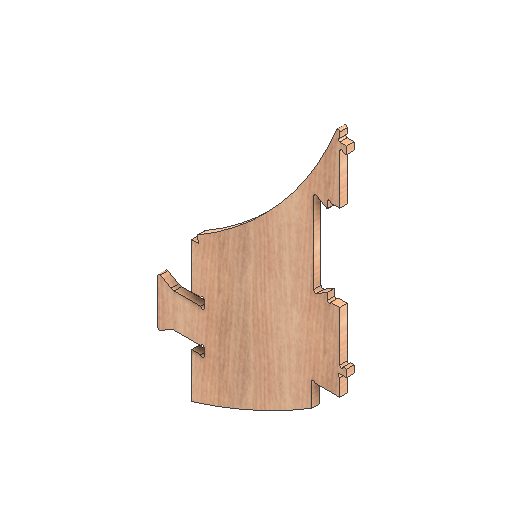
# Autodesk Inventor part: Support B
Saved by Autodesk Inventor 2021 (Build 250183000, 183)
## iProperties
Created: 2020-05-09
Part Number: Support B
Material: Wood (Birch)
Document SubType Name: Modeling
Designer: Dan Wikman
Density: 0.55 g/cm^3
Appearance: Birch - Natural Polished
Mass: 1422.74 g
Surface Area: 3324.08 cm^2
Volume: 2586.8 cm^3
Autodesk Inventor part; units mm, degrees
ref_plane "YZ Plane" through (0, 0, 0) normal (1, 0, 0) x (0, 1, 0)
ref_plane "XZ Plane" through (0, 0, 0) normal (0, 1, 0) x (-1, 0, 0)
ref_plane "XY Plane" through (0, 0, 0) normal (0, 0, 1) x (1, 0, 0)
sketch "CONTOURS" plane through (0, 0, 0) normal (0, 0, 1) x (1, 0, 0)
  line L0 (2379.4087, 421.1241) -> (2379.4087, 437.5136)
  line L1 (2083.0497, 275.5979) -> (2083.0497, 256.5979)
  arc A0 (2075.0497, 256.5979) -> (2083.0497, 256.5979) centre (2079.0497, 256.5979) ccw
  line L2 (2075.0497, 256.5979) -> (2051.9087, 256.5979)
  line L3 (2051.9087, 256.5979) -> (2010.928, 256.5979)
  arc A1 (2003.428, 258.6076) -> (2010.928, 256.5979) centre (2010.928, 271.5979) ccw
  line L4 (2003.428, 258.6076) -> (1977.9087, 273.3411)
  arc A2 (1977.9087, 273.3411) -> (1971.9087, 269.877) centre (1975.9087, 269.877) ccw
  line L5 (1971.9087, 269.877) -> (1971.9087, 161.3189)
  arc A3 (1971.9087, 161.3189) -> (1977.9087, 157.8548) centre (1975.9087, 161.3189) ccw
  line L6 (1977.9087, 157.8548) -> (2003.428, 172.5883)
  arc A4 (2010.928, 174.5979) -> (2003.428, 172.5883) centre (2010.928, 159.5979) ccw
  line L7 (2010.928, 174.5979) -> (2051.9087, 174.5979)
  line L8 (2051.9087, 174.5979) -> (2075.0497, 174.5979)
  arc A5 (2083.0497, 174.5979) -> (2075.0497, 174.5979) centre (2079.0497, 174.5979) ccw
  line L9 (2083.0497, 174.5979) -> (2083.0497, 155.5979)
  arc A6 (2075.0497, 155.5979) -> (2083.0497, 155.5979) centre (2079.0497, 155.5979) ccw
  line L10 (2075.0497, 155.5979) -> (2053.0497, 155.5979)
  line L11 (2053.0497, 155.5979) -> (2053.0497, 46.9498)
  arc A7 (2053.0497, 46.9498) -> (2341.9087, 177.362) centre (1668.415, 1284.0168) ccw
  line L12 (2341.9087, 177.362) -> (2341.9087, 234.1241)
  arc A8 (2349.9087, 234.1241) -> (2341.9087, 234.1241) centre (2345.9087, 234.1241) ccw
  line L13 (2349.9087, 234.1241) -> (2409.4087, 234.1241)
  line L14 (2409.4087, 234.1241) -> (2409.4087, 275.172)
  arc A9 (2409.4087, 283.172) -> (2409.4087, 275.172) centre (2409.4087, 279.172) ccw
  line L15 (2409.4087, 283.172) -> (2425.9087, 283.172)
  line L16 (2425.9087, 283.172) -> (2425.9087, 301.172)
  line L17 (2425.9087, 301.172) -> (2417.4087, 301.172)
  arc A10 (2409.4087, 301.172) -> (2417.4087, 301.172) centre (2413.4087, 301.172) ccw
  line L18 (2409.4087, 301.172) -> (2409.4087, 421.1241)
  line L19 (2409.4087, 421.1241) -> (2387.4087, 421.1241)
  arc A11 (2379.4087, 421.1241) -> (2387.4087, 421.1241) centre (2383.4087, 421.1241) ccw
  line L20 (2379.4087, 437.5136) -> (2379.1671, 437.3833)
  line L21 (2379.1671, 437.3833) -> (2378.928, 437.2484)
  line L22 (2378.928, 437.2484) -> (2353.7677, 422.7221)
  arc A12 (2346.2677, 427.0523) -> (2353.7677, 422.7221) centre (2351.2677, 427.0523) ccw
  line L23 (2346.2677, 427.0523) -> (2346.2677, 622.1959)
  arc A13 (2353.7677, 626.526) -> (2346.2677, 622.1959) centre (2351.2677, 622.1959) ccw
  line L24 (2353.7677, 626.526) -> (2378.928, 611.9997)
  line L25 (2378.928, 611.9997) -> (2379.1671, 611.8648)
  line L26 (2379.1671, 611.8648) -> (2379.4087, 611.7346)
  line L27 (2379.4087, 611.7346) -> (2379.4087, 628.1241)
  arc A14 (2387.4087, 628.1241) -> (2379.4087, 628.1241) centre (2383.4087, 628.1241) ccw
  line L28 (2387.4087, 628.1241) -> (2409.4087, 628.1241)
  line L29 (2409.4087, 628.1241) -> (2409.4087, 748.0761)
  arc A15 (2417.4087, 748.0761) -> (2409.4087, 748.0761) centre (2413.4087, 748.0761) ccw
  line L30 (2417.4087, 748.0761) -> (2425.9087, 748.0761)
  line L31 (2425.9087, 748.0761) -> (2425.9087, 766.0761)
  line L32 (2425.9087, 766.0761) -> (2409.4087, 766.0761)
  arc A16 (2409.4087, 774.0761) -> (2409.4087, 766.0761) centre (2409.4087, 770.0761) ccw
  line L33 (2409.4087, 774.0761) -> (2409.4087, 786.8861)
  arc A17 (2409.4087, 786.8861) -> (2401.6988, 788.3816) centre (2405.4087, 786.8861) ccw
  arc A18 (2066.9087, 401.2195) -> (2401.6988, 788.3816) centre (1668.7587, 1083.8435) ccw
  line L34 (2066.9087, 401.2195) -> (2066.9087, 392.5981)
  arc A19 (2066.9087, 384.5981) -> (2066.9087, 392.5981) centre (2066.9087, 388.5981) ccw
  line L35 (2066.9087, 384.5981) -> (2053.0497, 384.5981)
  line L36 (2053.0497, 384.5981) -> (2053.0497, 275.5979)
  line L37 (2053.0497, 275.5979) -> (2075.0497, 275.5979)
  arc A20 (2083.0497, 275.5979) -> (2075.0497, 275.5979) centre (2079.0497, 275.5979) ccw
  constraints: 76 end point, 42 point on circle, 21 centre point
sketch "HOLES" plane through (0, 0, 0) normal (0, 0, 1) x (1, 0, 0)
  arc A0 (2359.9087, 385.1025) -> (2355.9087, 381.1025) centre (2359.9087, 381.1025) ccw
  line L0 (2359.9087, 385.1025) -> (2389.9087, 385.1025)
  arc A1 (2393.9087, 381.1025) -> (2389.9087, 385.1025) centre (2389.9087, 381.1025) ccw
  line L1 (2393.9087, 381.1025) -> (2393.9087, 370.1025)
  arc A2 (2389.9087, 366.1025) -> (2393.9087, 370.1025) centre (2389.9087, 370.1025) ccw
  line L2 (2389.9087, 366.1025) -> (2359.9087, 366.1025)
  arc A3 (2355.9087, 370.1025) -> (2359.9087, 366.1025) centre (2359.9087, 370.1025) ccw
  line L3 (2355.9087, 370.1025) -> (2355.9087, 381.1025)
  constraints: 8 end point, 8 point on circle, 4 centre point
sketch "LETTERS" plane through (0, 0, 0) normal (0, 0, 1) x (1, 0, 0)
  arc A0 (2211.6565, 303.9645) -> (2200.9951, 304.2164) centre (2206.3294, 304.2452) ccw
  line L0 (2200.9964, 295.3379) -> (2200.9964, 303.7395)
  arc A1 (2200.9964, 303.7395) -> (2191.9817, 303.7395) centre (2196.489, 303.7395) ccw
  line L1 (2191.9817, 303.7395) -> (2191.9817, 295.3379)
  line L2 (2211.6565, 295.3379) -> (2211.6565, 299.2505)
  line L3 (2211.6565, 299.2505) -> (2211.6639, 304.2373)
  line L4 (2191.9817, 295.3379) -> (2211.6565, 295.3379)
  constraints: 10 end point, 5 point on circle, 3 tangent, 2 centre point, 1 point on line
extrude "Extrusion3" add sketch "CONTOURS" along normal blind 18
body "Solid1"
